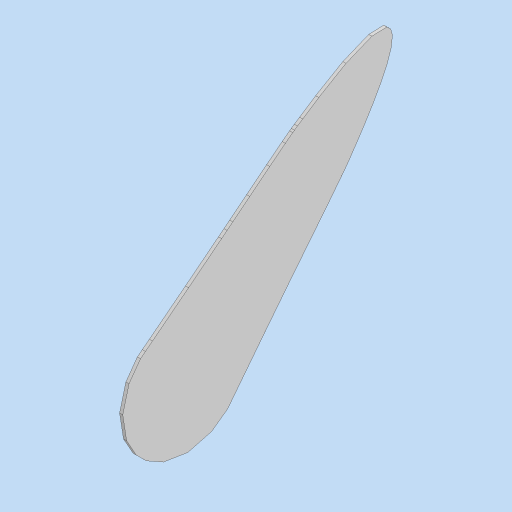
# Autodesk Inventor part: Sticker7
Saved by Autodesk Inventor 2024 (Build 280153000, 153)
## iProperties
Created: 2025-01-25
Part Number: Sticker7
Material: Generic
Document SubType Name: Modeling
Designer: Dmitry
Density: 1 g/cm^3
Appearance: Default
Author: Dmitry
Autodesk Inventor part; units mm, degrees
ref_plane "YZ Plane" through (0, 0, 0) normal (1, 0, 0) x (0, 1, 0)
ref_plane "XZ Plane" through (0, 0, 0) normal (0, 1, 0) x (-1, 0, 0)
ref_plane "XY Plane" through (0, 0, 0) normal (0, 0, 1) x (1, 0, 0)
sketch "Sketch1" plane through (0, 0, 0) normal (1, 0, 0) x (0, 1, 0)
  line L0 (11.5153, 6.5399) -> (13.2626, 6.1589)
  line L1 (-9.5192, 15.3385) -> (-9.5235, 15.3385)
  line L2 (-9.5235, 15.3385) -> (-9.5593, 15.3004)
  line L3 (-9.5593, 15.3004) -> (-9.5621, 15.2978)
  line L4 (-9.5621, 15.2978) -> (-9.9203, 14.9422)
  line L5 (-9.9203, 14.9422) -> (-10.6894, 13.5732)
  line L6 (-10.6894, 13.5732) -> (-10.9995, 11.6224)
  line L7 (-10.9995, 11.6224) -> (-10.4963, 9.7251)
  line L8 (-10.4963, 9.7251) -> (-9.5812, 8.4551)
  line L9 (-9.5812, 8.4551) -> (-9.1857, 8.1477)
  line L10 (-9.1857, 8.1477) -> (-8.6264, 7.7134)
  line L11 (-8.6264, 7.7134) -> (-5.7531, 5.4731)
  line L12 (-5.7531, 5.4731) -> (-3.125, 3.403)
  line L13 (-3.125, 3.403) -> (-2.6869, 3.0525)
  line L14 (-2.6869, 3.0525) -> (-2.235, 2.6918)
  line L15 (-2.235, 2.6918) -> (-0.8776, 1.6047)
  line L16 (-0.8776, 1.6047) -> (0.7277, 0.3271)
  line L17 (0.7277, 0.3271) -> (1.9751, -0.6483)
  line L18 (1.9751, -0.6483) -> (2.5659, -1.1004)
  line L19 (2.5659, -1.1004) -> (2.7096, -1.1969)
  line L20 (2.7096, -1.1969) -> (2.9464, -1.3595)
  line L21 (2.9464, -1.3595) -> (3.1338, -1.4865)
  line L22 (3.1338, -1.4865) -> (3.7002, -1.87)
  line L23 (3.7002, -1.87) -> (4.6441, -2.4873)
  line L24 (4.6441, -2.4873) -> (5.7068, -3.1426)
  line L25 (5.7068, -3.1426) -> (6.8158, -3.7623)
  line L26 (6.8158, -3.7623) -> (7.8978, -4.2754)
  line L27 (7.8978, -4.2754) -> (8.8818, -4.6132)
  line L28 (8.8818, -4.6132) -> (9.6959, -4.7021)
  line L29 (9.6959, -4.7021) -> (10.1645, -4.5726)
  line L30 (10.1645, -4.5726) -> (10.2664, -4.4735)
  line L31 (10.2664, -4.4735) -> (10.2776, -4.4608)
  line L32 (10.2776, -4.4608) -> (10.4693, -4.2627)
  line L33 (10.4693, -4.2627) -> (10.4289, -3.0664)
  line L34 (10.4289, -3.0664) -> (9.5831, -0.9963)
  line L35 (9.5831, -0.9963) -> (8.3108, 1.1754)
  line L36 (8.3108, 1.1754) -> (7.4706, 2.453)
  line L37 (7.4706, 2.453) -> (7.1838, 2.8747)
  line L38 (7.1838, 2.8747) -> (7.0213, 3.1134)
  line L39 (7.0213, 3.1134) -> (6.9248, 3.2557)
  line L40 (6.9248, 3.2557) -> (6.4739, 3.845)
  line L41 (6.4739, 3.845) -> (5.5001, 5.087)
  line L42 (5.5001, 5.087) -> (4.2278, 6.6872)
  line L43 (4.2278, 6.6872) -> (3.145, 8.041)
  line L44 (3.145, 8.041) -> (2.7851, 8.4906)
  line L45 (2.7851, 8.4906) -> (2.4351, 8.93)
  line L46 (2.4351, 8.93) -> (0.3586, 11.5615)
  line L47 (0.3586, 11.5615) -> (-1.8878, 14.4444)
  line L48 (-1.8878, 14.4444) -> (-2.3231, 15.0083)
  line L49 (-2.3231, 15.0083) -> (-2.6305, 15.402)
  line L50 (-2.6305, 15.402) -> (-3.9025, 16.3189)
  line L51 (-3.9025, 16.3189) -> (-5.8001, 16.8218)
  line L52 (-5.8001, 16.8218) -> (-7.7486, 16.5119)
  line L53 (-7.7486, 16.5119) -> (-9.1212, 15.7449)
  line L54 (-9.1212, 15.7449) -> (-9.475, 15.3842)
  line L55 (-9.475, 15.3842) -> (-9.4793, 15.3816)
  line L56 (-9.4793, 15.3816) -> (-9.5167, 15.3435)
  line L57 (-9.5167, 15.3435) -> (-9.5192, 15.3385)
  constraints: 116 end point
extrude "Extrusion27" add sketch "Sketch1" along normal blind 0.25
sketch "Sketch7" plane through (0, 0, 0) normal (-1, 0, 0) x (0, 0, 1)
  circle A0 centre (11.7567, -6.0872) radius 5
  circle A1 centre (11.7567, -6.0872) radius 0.5
  point P0 (0, 0)
  dimension "d91" = 10
  dimension "d92" = 1
  constraints: 2 centre point, 1 coincident
  measures "d91" diameter of A0
  measures "d92" diameter of A1
extrude "Extrusion30" [suppressed]
body "Solid6"
